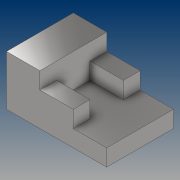
# Autodesk Inventor part: 46
Saved by Autodesk Inventor 2020.2 (Build 242310000, 310)
## iProperties
Created: 2020-09-17
Part Number: 46
Material: 鋼、碳鋼
Document SubType Name: Modeling
Designer: user
Density: 7.85 g/cm^3
Appearance: 半拋光
Mass: 345.4 g
Surface Area: 100 cm^2
Volume: 44 cm^3
Author: user
Autodesk Inventor part; units mm, degrees
ref_plane "YZ Plane" through (0, 0, 0) normal (1, 0, 0) x (0, 1, 0)
ref_plane "XZ Plane" through (0, 0, 0) normal (0, 1, 0) x (-1, 0, 0)
ref_plane "XY Plane" through (0, 0, 0) normal (0, 0, 1) x (1, 0, 0)
sketch "草圖1" plane through (0, 0, 0) normal (0, 1, 0) x (-1, 0, 0)
  line L0 (0, -20) -> (-60, -20)
  line L1 (-60, -20) -> (-60, 20)
  line L2 (-60, 20) -> (0, 20)
  line L3 (0, 20) -> (0, -20)
  point P0 (0, 0)
  point P1 (0, 0)
  dimension "d0" = 40
  dimension "d1" = 60
  constraints: 8 end point, 2 parallel, 1 coincident, 1 horizontal, 1 midpoint, 1 perpendicular
  measures "d0" distance of L2.end L0.start
  measures "d1" distance of L0.start L0.end
extrude "擠出1" add sketch "草圖1" along normal blind 30
sketch "草圖2" plane through (0, 0, 20) normal (0, 0, 1) x (1, 0, 0)
  line L0 (0, 0) -> (0, 30) projected
  line L1 (0, 30) -> (60, 30) projected
  line L2 (60, 30) -> (60, 0) projected
  line L3 (60, 0) -> (0, 0) projected
  line L4 (60, 30) -> (0, 30) projected
  line L5 (20, 30) -> (20, 20)
  line L6 (20, 20) -> (40, 20)
  line L7 (40, 20) -> (40, 10)
  line L8 (40, 10) -> (60, 10)
  point P0 (20, 30)
  dimension "d4" = 20
  dimension "d5" = 10
  dimension "d6" = 20
  dimension "d7" = 10
  constraints: 8 end point, 4 perpendicular, 2 point on line
  measures "d4" distance between parallel lines of L0 L5
  measures "d5" distance between parallel lines of L3 L8
  measures "d6" distance between parallel lines of L2 L7
  measures "d7" distance between parallel lines of L1 L6
extrude "擠出2" cut sketch "草圖2" against normal through all contours L1 L2 L8 L7 L6 L5
sketch "草圖3" plane through (20, 20, 20) normal (0, 1, 0) x (1, 0, 0)
  line L0 (0, 40) -> (0, 0) projected
  line L1 (20, 0) -> (0, 0) projected
  line L2 (20, 40) -> (20, 0) projected
  line L3 (0, 40) -> (20, 40) projected
  line L4 (-20, 40) -> (0, 40) projected
  line L5 (-20, 0) -> (-20, 40) projected
  line L6 (0, 0) -> (-20, 0) projected
  line L7 (0, 30) -> (20, 30)
  line L8 (20, 30) -> (20, 10)
  line L9 (20, 10) -> (0, 10)
  line L10 (0, 10) -> (0, 30)
  line L11 (20, 0) -> (20, 40) projected
  point P0 (-20, 20)
  point P1 (0, 20)
  point P2 (0, 10)
  point P3 (20, 10)
  point P4 (0, 30)
  dimension "d10" = 20
  constraints: 8 end point, 2 midpoint, 2 parallel, 1 collinear, 1 horizontal, 1 perpendicular
  measures "d10" distance between parallel lines of L9 L7
extrude "擠出3" cut sketch "草圖3" against normal blind 10 contours L7 L2 L9 L0
